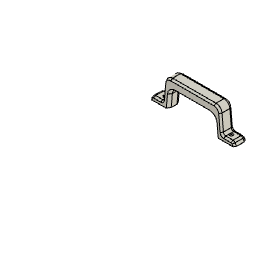
Griff_v56 (Autodesk Fusion 360 design; units mm, degrees)
Autodesk Fusion 360 part; units mm, degrees
note: some values were not read from the file. Set by a fixed rule: which sketch regions a step uses.
sketch "Skizze1" plane through (0, 0, 0) normal (0, 1, 0) x (1, 0, 0)
  line L0 (70, -154) -> (-70, -154)
  line L1 (70, -154) -> (66.5359, -160)
  line L2 (66.5359, -160) -> (48.5359, -160)
  line L3 (48.5359, -160) -> (45.1238, -199)
  line L4 (45.1238, -199) -> (0, -199)
  line L5 (0, -199) -> (0, -184) construction
  line L6 (0, -184) -> (37.3753, -184)
  line L7 (0, -184) -> (-37.3753, -184)
  line L8 (-45.1238, -199) -> (0, -199)
  line L9 (-48.5359, -160) -> (-45.1238, -199)
  line L10 (-66.5359, -160) -> (-48.5359, -160)
  line L11 (-70, -154) -> (-66.5359, -160)
  line L12 (37.3753, -184) -> (40, -154)
  line L13 (-37.3753, -184) -> (-40, -154)
  dimension "d611" = 6
  dimension "d612" = 60
  dimension "d613" = 30
  dimension "d614" = 15
  dimension "d615" = 95
  dimension "d616" = 18
  dimension "d633" = 80
  constraint coincident L0.start L1.start
  constraint parallel L0 L2
  constraint parallel L2 L4
  constraint perpendicular L2 L5
  constraint perpendicular L5 L6
  constraint symmetric L0.start L5 L0.end
  constraint symmetric L1.end L5 L10.start
  constraint symmetric L2.end L5 L9.start
  constraint symmetric L3.end L5 L8.start
  constraint symmetric L4.end L5 L8.end
  constraint symmetric L6.start L5 L7.start
  constraint symmetric L5 L6.end L7.end
  constraint vertical origin L5.end
  constraint coincident L0 L12.end
  constraint symmetric L5 L12.end L13.end
  constraint parallel L3 L12
  measures "d611" distance of L0 L2
  measures "d612" angle of L0 L1
  measures "d613" distance of L0 L6
  measures "d614" distance of L4 L6
  measures "d615" angle of L2 L3
  measures "d616" distance of L1.end L2.end
  measures "d633" distance of L12.end L13.end
extrude "Extrusion1" add sketch "Skizze1" along normal mid plane 20 contours L0 L1 L2 L3 L4 L6 L7 L8 L9 L10 L11 L12 L13
sketch "Skizze2" plane through (0, 0, 160) normal (0, 0, 1) x (-1, 0, 0)
  line L0 (-66.5359, 10) -> (-66.5359, -10)
  line L1 (-66.5359, -10) -> (-48.5359, -10)
  line L2 (-48.5359, -10) -> (-48.5359, 10)
  line L3 (-48.5359, 10) -> (-66.5359, 10)
  line L4 (70, 73.2) -> (70, -73.2)
  line L5 (-70, -73.2) -> (-70, 73.2)
  point P0 (55, 0)
  point P1 (-55, 0)
  dimension "d619" = 15
  dimension "d620" = 15
  constraint horizontal origin P0
  constraint horizontal origin P1
  measures "d619" distance of P0 L4
  measures "d620" distance of P1 L5
hole "Bohrung1" at (-55, 0, 160) at (55, 0, 160) direction (0, 0, -1) diameter 3.4 depth 6.9 tip angle 180 countersink diameter 5.5 countersink angle 90
fillet "Abrundung1" radius 10 4 edges at (45.1238, 0, 199) (-45.1238, 0, 199) (-37.3753, 0, 184) (37.3753, 0, 184)
fillet "Abrundung1" radius 4 4 edges at (66.5359, 0, 160) (-66.5359, 0, 160) (48.5359, 0, 160) (-48.5359, 0, 160)
chamfer "Fase1" distance 2 angle 60 26 edges at (-68.8453, 10, 156) (-66.2265, 10, 159.4641) (-58.2139, 10, 160) (-49.4989, 10, 161.0509) (-47.0695, 10, 176.7615) (-42.7164, 10, 196.3728) (0, 10, 199) (42.7164, 10, 196.3728) (47.0695, 10, 176.7615) (49.4989, 10, 161.0509) (58.2139, 10, 160) (66.2265, 10, 159.4641) (68.8453, 10, 156) (68.8453, -10, 156) (66.2265, -10, 159.4641) (58.2139, -10, 160) (49.4989, -10, 161.0509) (47.0695, -10, 176.7615) (42.7164, -10, 196.3728) (0, -10, 199) (-42.7164, -10, 196.3728) (-47.0695, -10, 176.7615) (-49.4989, -10, 161.0509) (-58.2139, -10, 160) (-66.2265, -10, 159.4641) (-68.8453, -10, 156) measured on face at (9.404, 10, 194) measured on face at (-67.09, 3.3333, 158.7929) measured on face at (9.404, 10, 194) measured on face at (-48.5711, 3.3333, 162.3201) measured on face at (9.404, 10, 194) measured on face at (-36.4548, 3.3333, 198.9878) measured on face at (9.404, 10, 194) measured on face at (45.8672, 3.3333, 190.3629) measured on face at (9.404, 10, 194) measured on face at (48.5711, 3.3333, 162.3201) measured on face at (9.404, 10, 194) measured on face at (67.09, 3.3333, 158.7929) measured on face at (9.404, 10, 194) measured on face at (9.404, -10, 194) measured on face at (67.09, 3.3333, 158.7929) measured on face at (9.404, -10, 194) measured on face at (48.5711, 3.3333, 162.3201) measured on face at (9.404, -10, 194) measured on face at (45.8672, 3.3333, 190.3629) measured on face at (9.404, -10, 194) measured on face at (-36.4548, 3.3333, 198.9878) measured on face at (9.404, -10, 194) measured on face at (-48.5711, 3.3333, 162.3201) measured on face at (9.404, -10, 194) measured on face at (-67.09, 3.3333, 158.7929) measured on face at (9.404, -10, 194)
chamfer "Fase2" distance 3 angle 60 10 edges at (39.087, 10, 164.4358) (34.9679, 10, 181.3728) (0, 10, 184) (-34.9679, 10, 181.3728) (-39.087, 10, 164.4358) (-39.087, -10, 164.4358) (-34.9679, -10, 181.3728) (0, -10, 184) (34.9679, -10, 181.3728) (39.087, -10, 164.4358) measured on face at (9.404, 10, 192.6667) measured on face at (28.7063, -3.3333, 183.9878) measured on face at (9.404, 10, 192.6667) measured on face at (-38.0392, -3.3333, 175.8509) measured on face at (9.404, 10, 192.6667) measured on face at (-9.404, -10, 192.6667) measured on face at (-38.0392, -3.3333, 175.8509) measured on face at (-9.404, -10, 192.6667) measured on face at (28.7063, -3.3333, 183.9878) measured on face at (-9.404, -10, 192.6667)
equation "d620 = d619"
